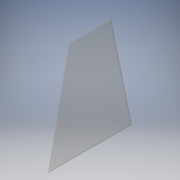
# Autodesk Inventor part: Polycarb Front Pannel
Saved by Autodesk Inventor 2016 (Build 200138000, 138)
## iProperties
Created: 2018-05-16
Part Number: Polycarb Front Pannel
Material: Polycarbonate, Clear
Document SubType Name: Modeling
Designer: Kade
Density: 1.2 g/cm^3
Appearance: Polycarbonate - Clear
Mass: 1068.25 g
Surface Area: 5685.53 cm^2
Volume: 890.211 cm^3
Author: Kade
Autodesk Inventor part; units mm, degrees
ref_plane "YZ Plane" through (0, 0, 0) normal (1, 0, 0) x (0, 1, 0)
ref_plane "XZ Plane" through (0, 0, 0) normal (0, 1, 0) x (-1, 0, 0)
ref_plane "XY Plane" through (0, 0, 0) normal (0, 0, 1) x (1, 0, 0)
sketch "Sketch1" plane through (0, 0, 0) normal (1, 0, 0) x (0, 1, 0)
  line L0 (0, 0) -> (0, 406.4)
  line L1 (0, 0) -> (0, 203.2)
  line L2 (0, 203.2) -> (457.2, 203.2) construction
  line L3 (497.7363, 304.8) -> (497.7363, 101.6)
  line L4 (497.7363, 304.8) -> (0, 406.4)
  line L5 (497.7363, 101.6) -> (0, 0)
  dimension "d0" = 406.4
  dimension "d4" = 203.2
  dimension "d5" = 203.2
  dimension "d11" = 101.6
  dimension "d12" = 101.6
  dimension "d14" = 508
  dimension "d15" = 497.7363
  constraints: 12 end point, 1 horizontal, 1 midpoint, 1 parallel, 1 vertical
  measures "d0" distance of L0.start L0.end
  measures "d4" distance of L3.start L3.end
  measures "d5" distance from line of L0.start L2
  measures "d11" vertical distance of L0.start L3.end
  measures "d12" vertical distance of L0.end L3.start
  measures "d14" distance of L3.end L0.start
  measures "d15" distance between parallel lines of L0 L3
extrude "Extrusion1" add sketch "Sketch1" along normal blind 3.175
body "Solid1"
